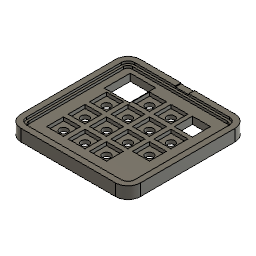
OpenMicroSolderTool (Autodesk Fusion 360 design; units mm, degrees)
Autodesk Fusion 360 part; units mm, degrees
sketch "Sketch1" plane through (0, 0, 0) normal (0, 1, 0) x (1, 0, 0)
  line L0 (0, 0) -> (0, 32) construction
  line L1 (0, 0) -> (-33, 0) construction
  line L2 (-42, 53) -> (42, 53)
  line L3 (53, 42) -> (53, -42)
  line L4 (42, -53) -> (-42, -53)
  line L5 (-53, -42) -> (-53, 42)
  arc A0 (-42, 53) -> (-53, 42) centre (-42, 42) ccw
  arc A1 (-53, -42) -> (-42, -53) centre (-42, -42) ccw
  arc A2 (42, -53) -> (53, -42) centre (42, -42) ccw
  arc A3 (53, 42) -> (42, 53) centre (42, 42) ccw
  point P0 (-53, 53)
  point P1 (53, 53)
  dimension "d1" = 106
  dimension "d2" = 11
  dimension "d49" = 106
  constraint coincident L0.start L1.start
  constraint vertical L0
  constraint perpendicular L0 L1
  constraint horizontal L2
  constraint vertical L3
  constraint horizontal L4
  constraint vertical L5
  constraint symmetric L0 L3 L5
  constraint symmetric L1 L2 L4
  constraint coincident P0 L2
  constraint coincident P0 L5
  constraint tangent L2 A0
  constraint tangent L5 A0
  constraint tangent L4 A1
  constraint tangent L5 A1
  constraint equal A0 A1
  constraint tangent L3 A2
  constraint tangent L4 A2
  constraint equal A0 A2
  constraint coincident P1 L2
  constraint coincident P1 L3
  constraint tangent L2 A3
  constraint tangent L3 A3
  constraint equal A0 A3
  measures "d1" distance of P0 P1
  measures "d2" radius of A0
  measures "d49" distance of L2 L4
extrude "Extrude1" add sketch "Sketch1" along normal blind 10.6
sketch "Sketch2" plane through (0, 10.6, 0) normal (0, 1, 0) x (-1, 0, 0)
  arc A0 (-42, 53) -> (-53, 42) centre (-42, 42) ccw
  line L0 (-53, 42) -> (-53, -42)
  arc A1 (-53, -42) -> (-42, -53) centre (-42, -42) ccw
  line L1 (-42, -53) -> (42, -53)
  arc A2 (42, -53) -> (53, -42) centre (42, -42) ccw
  line L2 (53, -42) -> (53, 42)
  arc A3 (53, 42) -> (42, 53) centre (42, 42) ccw
  line L3 (42, 53) -> (-42, 53)
  line L4 (48, -42) -> (48, 42)
  arc A4 (48, 42) -> (42, 48) centre (42, 42) ccw
  line L5 (42, 48) -> (-42, 48)
  arc A5 (-42, 48) -> (-48, 42) centre (-42, 42) ccw
  line L6 (-48, 42) -> (-48, -42)
  arc A6 (-48, -42) -> (-42, -48) centre (-42, -42) ccw
  line L7 (-42, -48) -> (42, -48)
  arc A7 (42, -48) -> (48, -42) centre (42, -42) ccw
  dimension "d5" = -5
extrude "Extrude2" cut sketch "Sketch2" against normal blind 2 contours L4 A4 L5 A5 L6 A6 L7 A7
sketch "Sketch3" plane through (0, 8.6, 0) normal (0, 1, 0) x (-1, 0, 0)
  arc A0 (42, -48) -> (48, -42) centre (42, -42) ccw
  line L0 (48, -42) -> (48, 42)
  arc A1 (48, 42) -> (42, 48) centre (42, 42) ccw
  line L1 (42, 48) -> (-42, 48)
  arc A2 (-42, 48) -> (-48, 42) centre (-42, 42) ccw
  line L2 (-48, 42) -> (-48, -42)
  arc A3 (-48, -42) -> (-42, -48) centre (-42, -42) ccw
  line L3 (-42, -48) -> (42, -48)
  line L4 (46, -42) -> (46, 42)
  arc A4 (46, 42) -> (42, 46) centre (42, 42) ccw
  line L5 (42, 46) -> (-42, 46)
  arc A5 (-42, 46) -> (-46, 42) centre (-42, 42) ccw
  line L6 (-46, 42) -> (-46, -42)
  arc A6 (-46, -42) -> (-42, -46) centre (-42, -42) ccw
  line L7 (-42, -46) -> (42, -46)
  arc A7 (42, -46) -> (46, -42) centre (42, -42) ccw
  dimension "d8" = -2
extrude "Extrude3" cut sketch "Sketch3" against normal blind 2.2 contours L4 A4 L5 A5 L6 A6 L7 A7
sketch "Sketch5" plane through (0, 6.4, 0) normal (0, 1, 0) x (-1, 0, 0)
  arc A0 (42, -46) -> (46, -42) centre (42, -42) ccw
  line L0 (46, -42) -> (46, 42)
  arc A1 (46, 42) -> (42, 46) centre (42, 42) ccw
  line L1 (42, 46) -> (-42, 46)
  arc A2 (-42, 46) -> (-46, 42) centre (-42, 42) ccw
  line L2 (-46, 42) -> (-46, -42)
  arc A3 (-46, -42) -> (-42, -46) centre (-42, -42) ccw
  line L3 (-42, -46) -> (42, -46)
  line L4 (0, 0) -> (0, -26) construction
  line L5 (0, 0) -> (25, 0) construction
  line L6 (-2.025, -36.075) -> (-17.025, -36.075)
  line L7 (-17.025, -36.075) -> (-17.025, -21.075)
  line L8 (-17.025, -21.075) -> (-2.025, -21.075)
  line L9 (-2.025, -21.075) -> (-2.025, -36.075)
  line L10 (17.025, -36.075) -> (2.025, -36.075)
  line L11 (2.025, -36.075) -> (2.025, -21.075)
  line L12 (2.025, -21.075) -> (17.025, -21.075)
  line L13 (17.025, -21.075) -> (17.025, -36.075)
  line L14 (-21.075, -17.025) -> (-36.075, -17.025)
  line L15 (-36.075, -17.025) -> (-36.075, -2.025)
  line L16 (-36.075, -2.025) -> (-21.075, -2.025)
  line L17 (-21.075, -2.025) -> (-21.075, -17.025)
  line L18 (-2.025, -17.025) -> (-17.025, -17.025)
  line L19 (-17.025, -17.025) -> (-17.025, -2.025)
  line L20 (-17.025, -2.025) -> (-2.025, -2.025)
  line L21 (-2.025, -2.025) -> (-2.025, -17.025)
  line L22 (17.025, -17.025) -> (2.025, -17.025)
  line L23 (2.025, -17.025) -> (2.025, -2.025)
  line L24 (2.025, -2.025) -> (17.025, -2.025)
  line L25 (17.025, -2.025) -> (17.025, -17.025)
  line L26 (36.0775, -17.025) -> (21.0775, -17.025)
  line L27 (21.0775, -17.025) -> (21.0775, -2.025)
  line L28 (21.0775, -2.025) -> (36.0775, -2.025)
  line L29 (36.0775, -2.025) -> (36.0775, -17.025)
  line L30 (-21.075, 2.025) -> (-36.075, 2.025)
  line L31 (-36.075, 2.025) -> (-36.075, 17.025)
  line L32 (-36.075, 17.025) -> (-21.075, 17.025)
  line L33 (-21.075, 17.025) -> (-21.075, 2.025)
  line L34 (-2.025, 2.025) -> (-17.025, 2.025)
  line L35 (-17.025, 2.025) -> (-17.025, 17.025)
  line L36 (-17.025, 17.025) -> (-2.025, 17.025)
  line L37 (-2.025, 17.025) -> (-2.025, 2.025)
  line L38 (17.025, 2.025) -> (2.025, 2.025)
  line L39 (2.025, 2.025) -> (2.025, 17.025)
  line L40 (2.025, 17.025) -> (17.025, 17.025)
  line L41 (17.025, 17.025) -> (17.025, 2.025)
  line L42 (36.0775, 2.025) -> (21.0775, 2.025)
  line L43 (21.0775, 2.025) -> (21.0775, 17.025)
  line L44 (21.0775, 17.025) -> (36.0775, 17.025)
  line L45 (36.0775, 17.025) -> (36.0775, 2.025)
  line L46 (36.0775, 21.075) -> (21.0775, 21.075)
  line L47 (21.0775, 21.075) -> (21.0775, 36.075)
  line L48 (21.0775, 36.075) -> (36.0775, 36.075)
  line L49 (36.0775, 36.075) -> (36.0775, 21.075)
  line L50 (-2.025, 21.075) -> (-17.025, 21.075)
  line L51 (-17.025, 21.075) -> (-17.025, 36.075)
  line L52 (-17.025, 36.075) -> (-2.025, 36.075)
  line L53 (-2.025, 36.075) -> (-2.025, 21.075)
  line L54 (17.025, 21.075) -> (2.025, 21.075)
  line L55 (2.025, 21.075) -> (2.025, 36.075)
  line L56 (2.025, 36.075) -> (17.025, 36.075)
  line L57 (17.025, 36.075) -> (17.025, 21.075)
  line L58 (9.525, -36.075) -> (9.525, -21.075) construction
  line L59 (17.025, -28.575) -> (2.025, -28.575) construction
  line L60 (28.5775, -17.025) -> (28.5775, -2.025) construction
  line L61 (36.0775, -9.525) -> (21.0775, -9.525) construction
  line L62 (-2.025, 9.525) -> (-17.025, 9.525) construction
  line L63 (-9.525, 2.025) -> (-9.525, 17.025) construction
  line L64 (36.0775, 28.575) -> (21.0775, 28.575) construction
  dimension "d16" = 9.525
  dimension "d17" = 28.575
  dimension "d18" = 9.525
  dimension "d19" = 28.575
  dimension "d20" = 28.5775
  dimension "d21" = 9.525
  dimension "d23" = 15
  dimension "d24" = 9.525
  constraint coincident L4.start L5.start
  constraint vertical L4
  constraint perpendicular L4 L5
  constraint horizontal L6
  constraint vertical L7
  constraint horizontal L8
  constraint vertical L9
  constraint horizontal L10
  constraint vertical L11
  constraint horizontal L12
  constraint vertical L13
  constraint horizontal L14
  constraint vertical L15
  constraint horizontal L16
  constraint vertical L17
  constraint horizontal L18
  constraint vertical L19
  constraint horizontal L20
  constraint vertical L21
  constraint horizontal L22
  constraint vertical L23
  constraint horizontal L24
  constraint vertical L25
  constraint horizontal L26
  constraint vertical L27
  constraint horizontal L28
  constraint vertical L29
  constraint horizontal L30
  constraint vertical L31
  constraint horizontal L32
  constraint vertical L33
  constraint horizontal L34
  constraint vertical L35
  constraint horizontal L36
  constraint vertical L37
  constraint horizontal L38
  constraint vertical L39
  constraint horizontal L40
  constraint vertical L41
  constraint horizontal L42
  constraint vertical L43
  constraint horizontal L44
  constraint vertical L45
  constraint horizontal L46
  constraint vertical L47
  constraint horizontal L48
  constraint vertical L49
  constraint horizontal L50
  constraint vertical L51
  constraint horizontal L52
  constraint vertical L53
  constraint horizontal L54
  constraint vertical L55
  constraint horizontal L56
  constraint vertical L57
  constraint equal L10 L13
  constraint equal L6 L10
  constraint equal L6 L9
  constraint equal L6 L14
  constraint equal L14 L17
  constraint equal L17 L18
  constraint equal L18 L21
  constraint equal L21 L22
  constraint equal L22 L25
  constraint equal L26 L29
  constraint equal L22 L26
  constraint equal L29 L45
  constraint equal L42 L45
  constraint equal L38 L42
  constraint equal L38 L41
  constraint equal L34 L38
  constraint equal L34 L37
  constraint equal L30 L34
  constraint equal L30 L33
  constraint equal L33 L46
  constraint equal L46 L49
  constraint equal L46 L50
  constraint equal L49 L53
  constraint equal L50 L54
  constraint equal L54 L57
  constraint collinear L6 L10
  constraint collinear L22 L26
  constraint collinear L18 L22
  constraint collinear L14 L18
  constraint collinear L38 L42
  constraint collinear L34 L38
  constraint collinear L30 L34
  constraint collinear L50 L54
  constraint collinear L46 L50
  constraint collinear L29 L45
  constraint collinear L13 L25
  constraint collinear L25 L41
  constraint collinear L41 L57
  constraint collinear L9 L21
  constraint collinear L21 L37
  constraint collinear L37 L53
  constraint collinear L17 L33
  constraint midpoint L10 L58.start
  constraint midpoint L12 L58.end
  constraint midpoint L13 L59.start
  constraint midpoint L11 L59.end
  constraint midpoint L26 L60.start
  constraint midpoint L28 L60.end
  constraint midpoint L29 L61.start
  constraint midpoint L27 L61.end
  constraint midpoint L37 L62.start
  constraint midpoint L35 L62.end
  constraint midpoint L34 L63.start
  constraint midpoint L36 L63.end
  constraint midpoint L49 L64.start
  constraint midpoint L47 L64.end
  constraint collinear L45 L49
  measures "d16" distance of L4 L58
  measures "d17" distance of L5 L59
  measures "d18" distance of L5 L62
  measures "d19" distance of L5 L64
  measures "d20" distance of L4 L60
  measures "d21" distance of L4 L63
  measures "d23" distance of L6.end L7.end
  measures "d24" distance of L5 L61
extrude "Extrude5" cut sketch "Sketch5" against normal blind 3.1 contours L6 L7 L8 L9 | L10 L11 L12 L13 | L14 L15 L16 L17 | L18 L19 L20 L21 | L22 L23 L24 L25 | L26 L27 L28 L29 | L30 L31 L32 L33 | L34 L35 L36 L37 | L38 L39 L40 L41 | L42 L43 L44 L45 | L46 L47 L48 L49 | L50 L51 L52 L53 | L54 L55 L56 L57
sketch "Sketch6" plane through (0, 3.3, 0) normal (0, 1, 0) x (-1, 0, 0)
  line L0 (17.025, -21.075) -> (2.025, -21.075)
  line L1 (2.025, -21.075) -> (2.025, -36.075)
  line L2 (2.025, -36.075) -> (17.025, -36.075)
  line L3 (17.025, -36.075) -> (17.025, -21.075)
  line L4 (9.525, -36.075) -> (9.525, -21.075) construction
  line L5 (17.025, -28.575) -> (2.025, -28.575) construction
  circle A0 centre (9.525, -28.575) radius 3.5
  circle A1 centre (-9.525, -28.575) radius 3.5
  circle A2 centre (28.575, -9.525) radius 3.5
  circle A3 centre (9.525, -9.525) radius 3.5
  circle A4 centre (-9.525, -9.525) radius 3.5
  circle A5 centre (-28.575, -9.525) radius 3.5
  circle A6 centre (-28.575, 9.525) radius 3.5
  circle A7 centre (-9.525, 9.525) radius 3.5
  circle A8 centre (9.525, 9.525) radius 3.5
  circle A9 centre (28.575, 9.525) radius 3.5
  circle A10 centre (9.525, 28.575) radius 3.5
  circle A11 centre (-9.525, 28.575) radius 3.5
  circle A12 centre (28.575, 28.575) radius 3.5
  line L6 (46, -9.525) -> (-46, -9.525) construction
  line L7 (46, 9.525) -> (-46, 9.525) construction
  line L8 (28.575, -46) -> (28.575, 46) construction
  line L9 (-9.525, -46) -> (-9.525, 46) construction
  line L10 (-28.575, -46) -> (-28.575, 46) construction
  line L11 (46, 28.575) -> (-46, 28.575) construction
  line L12 (42, -46) -> (-42, -46)
  line L13 (-42, 46) -> (42, 46)
  line L14 (-46, -42) -> (-46, 42)
  line L15 (46, 42) -> (46, -42)
  dimension "d27" = 7
  dimension "d28" = 28.575
  dimension "d29" = 9.525
  dimension "d30" = 9.525
  dimension "d31" = 9.525
  dimension "d32" = 28.575
  dimension "d33" = 28.575
  constraint midpoint L2 L4.start
  constraint midpoint L0 L4.end
  constraint midpoint L3 L5.start
  constraint midpoint L1 L5.end
  constraint midpoint L5 A0.centre
  constraint horizontal L6
  constraint horizontal L7
  constraint vertical L8
  constraint vertical L9
  constraint perpendicular L7 L10
  constraint parallel L7 L11
  constraint coincident L8.start L12
  constraint coincident L8.end L13
  constraint coincident L9.start L12
  constraint coincident L9.end L13
  constraint coincident L10.start L12
  constraint coincident L10.end L13
  constraint coincident L11.end L14
  constraint coincident L7.end L14
  constraint coincident L6.end L14
  constraint coincident L6.start L15
  constraint coincident L7.start L15
  constraint coincident L11.start L15
  constraint equal A0 A1
  constraint equal A1 A4
  constraint equal A4 A5
  constraint equal A3 A4
  constraint equal A2 A3
  constraint equal A2 A9
  constraint equal A8 A9
  constraint equal A7 A8
  constraint equal A6 A7
  constraint equal A6 A12
  constraint equal A11 A12
  constraint equal A10 A11
  constraint coincident L5 A1.centre
  constraint coincident A1.centre L9
  constraint coincident A2.centre L8
  constraint coincident A2.centre L6
  constraint coincident A3.centre L6
  constraint coincident L4 A3.centre
  constraint coincident A4.centre L6
  constraint coincident A4.centre L9
  constraint coincident A5.centre L6
  constraint coincident A5.centre L10
  constraint coincident A6.centre L7
  constraint coincident A6.centre L10
  constraint coincident A7.centre L7
  constraint coincident A7.centre L9
  constraint coincident A8.centre L7
  constraint coincident L4 A8.centre
  constraint coincident A9.centre L8
  constraint coincident A9.centre L7
  constraint coincident A10.centre L11
  constraint coincident L4 A10.centre
  constraint coincident A11.centre L9
  constraint coincident A11.centre L11
  constraint coincident A12.centre L11
  constraint coincident A12.centre L8
  measures "d27" diameter of A0
  measures "d28" distance of origin L8
  measures "d29" distance of origin L9
  measures "d30" distance of origin L6
  measures "d31" distance of origin L7
  measures "d32" distance of origin L11
  measures "d33" distance of origin L10
extrude "Extrude6" cut sketch "Sketch6" against normal up to surface (3.3 mm away) contours A0 | A1 | A2 | A3 | A4 | A5 | A6 | A7 | A8 | A9 | A10 | A11 | A12
sketch "Sketch7" plane through (0, 6.4, 0) normal (0, 1, 0) x (-1, 0, 0)
  arc A0 (42, -46) -> (46, -42) centre (42, -42) ccw
  line L0 (46, -42) -> (46, 42)
  arc A1 (46, 42) -> (42, 46) centre (42, 42) ccw
  line L1 (42, 46) -> (-42, 46)
  arc A2 (-42, 46) -> (-46, 42) centre (-42, 42) ccw
  line L2 (-46, 42) -> (-46, -42)
  arc A3 (-46, -42) -> (-42, -46) centre (-42, -42) ccw
  line L3 (-42, -46) -> (42, -46)
  line L4 (21.0775, 21.075) -> (21.0775, 36.075)
  line L5 (21.0775, 36.075) -> (36.0775, 36.075)
  line L6 (36.0775, 36.075) -> (36.0775, 21.075)
  line L7 (36.0775, 21.075) -> (21.0775, 21.075)
  line L8 (2.025, 2.025) -> (2.025, 17.025)
  line L9 (2.025, 17.025) -> (17.025, 17.025)
  line L10 (17.025, 17.025) -> (17.025, 2.025)
  line L11 (17.025, 2.025) -> (2.025, 2.025)
  line L12 (-17.025, -17.025) -> (-17.025, -2.025)
  line L13 (-17.025, -2.025) -> (-2.025, -2.025)
  line L14 (-2.025, -2.025) -> (-2.025, -17.025)
  line L15 (-2.025, -17.025) -> (-17.025, -17.025)
  line L16 (2.025, -36.075) -> (2.025, -21.075)
  line L17 (2.025, -21.075) -> (17.025, -21.075)
  line L18 (17.025, -21.075) -> (17.025, -36.075)
  line L19 (17.025, -36.075) -> (2.025, -36.075)
  line L20 (2.025, -17.025) -> (2.025, -2.025)
  line L21 (2.025, -2.025) -> (17.025, -2.025)
  line L22 (17.025, -2.025) -> (17.025, -17.025)
  line L23 (17.025, -17.025) -> (2.025, -17.025)
  line L24 (-17.025, 2.025) -> (-17.025, 17.025)
  line L25 (-17.025, 17.025) -> (-2.025, 17.025)
  line L26 (-2.025, 17.025) -> (-2.025, 2.025)
  line L27 (-2.025, 2.025) -> (-17.025, 2.025)
  line L28 (-17.025, 21.075) -> (-17.025, 36.075)
  line L29 (-17.025, 36.075) -> (-2.025, 36.075)
  line L30 (-2.025, 36.075) -> (-2.025, 21.075)
  line L31 (-2.025, 21.075) -> (-17.025, 21.075)
  line L32 (21.0775, 2.025) -> (21.0775, 17.025)
  line L33 (21.0775, 17.025) -> (36.0775, 17.025)
  line L34 (36.0775, 17.025) -> (36.0775, 2.025)
  line L35 (36.0775, 2.025) -> (21.0775, 2.025)
  line L36 (-36.075, -17.025) -> (-36.075, -2.025)
  line L37 (-36.075, -2.025) -> (-21.075, -2.025)
  line L38 (-21.075, -2.025) -> (-21.075, -17.025)
  line L39 (-21.075, -17.025) -> (-36.075, -17.025)
  line L40 (-17.025, -36.075) -> (-17.025, -21.075)
  line L41 (-17.025, -21.075) -> (-2.025, -21.075)
  line L42 (-2.025, -21.075) -> (-2.025, -36.075)
  line L43 (-2.025, -36.075) -> (-17.025, -36.075)
  line L44 (21.0775, -17.025) -> (21.0775, -2.025)
  line L45 (21.0775, -2.025) -> (36.0775, -2.025)
  line L46 (36.0775, -2.025) -> (36.0775, -17.025)
  line L47 (36.0775, -17.025) -> (21.0775, -17.025)
  line L48 (-36.075, 2.025) -> (-36.075, 17.025)
  line L49 (-36.075, 17.025) -> (-21.075, 17.025)
  line L50 (-21.075, 17.025) -> (-21.075, 2.025)
  line L51 (-21.075, 2.025) -> (-36.075, 2.025)
  line L52 (2.025, 21.075) -> (2.025, 36.075)
  line L53 (2.025, 36.075) -> (17.025, 36.075)
  line L54 (17.025, 36.075) -> (17.025, 21.075)
  line L55 (17.025, 21.075) -> (2.025, 21.075)
  line L56 (-20.575, -36.575) -> (-36.575, -36.575)
  line L57 (-36.575, -36.575) -> (-36.575, -20.575)
  line L58 (-36.575, -20.575) -> (-20.575, -20.575)
  line L59 (-20.575, -20.575) -> (-20.575, -36.575)
  line L60 (40, -42) -> (17.625, -42)
  line L61 (17.625, -42) -> (17.625, -19.025)
  line L62 (17.625, -19.025) -> (40, -19.025)
  line L63 (40, -19.025) -> (40, -42)
  line L64 (-28.575, -36.575) -> (-28.575, -20.575) construction
  line L65 (-20.575, -28.575) -> (-36.575, -28.575) construction
  dimension "d36" = 16
  dimension "d37" = 4
  dimension "d40" = 28.575
  dimension "d43" = 6
  dimension "d44" = 28.575
  dimension "d50" = 0.6
  dimension "d54" = 2
  constraint horizontal L56
  constraint vertical L57
  constraint horizontal L58
  constraint vertical L59
  constraint equal L56 L59
  constraint horizontal L60
  constraint vertical L61
  constraint horizontal L62
  constraint vertical L63
  constraint midpoint L56 L64.start
  constraint midpoint L58 L64.end
  constraint midpoint L59 L65.start
  constraint midpoint L57 L65.end
  measures "d36" distance of L56.start L56.end
  measures "d37" distance of L3 L60
  measures "d40" distance of origin L65
  measures "d43" distance of L0 L63
  measures "d44" distance of origin L64
  measures "d50" distance of L18 L61
  measures "d54" distance of L47 L62
extrude "Extrude7" cut sketch "Sketch7" against normal up to surface (6.4 mm away) contours L56 L57 L58 L59 | L60 L61 L62 L63
sketch "Sketch8" plane through (0, 0, -53) normal (0, 0, -1) x (-1, 0, 0)
  line L0 (-42, 0) -> (42, 0)
  line L1 (42, 0) -> (42, 10.6)
  line L2 (42, 10.6) -> (-42, 10.6)
  line L3 (-42, 10.6) -> (-42, 0)
  line L4 (0, 0) -> (0, 10.6) construction
  line L5 (6, 10.6) -> (-6, 10.6)
  line L6 (-6, 10.6) -> (-6, 9.8)
  line L7 (-6, 9.8) -> (6, 9.8)
  line L8 (6, 9.8) -> (6, 10.6)
  dimension "d45" = 0.8
  dimension "d46" = 12
  constraint coincident L4.start origin
  constraint midpoint L2 L4.end
  constraint horizontal L5
  constraint vertical L6
  constraint horizontal L7
  constraint vertical L8
  constraint coincident L2 L5.start
  constraint symmetric L4 L6 L8
  measures "d45" distance of L5 L7
  measures "d46" distance of L6 L8
extrude "Extrude8" cut sketch "Sketch8" against normal up to surface (5 mm away) contours L2 L5 L6 L7 L8
